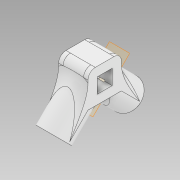
# Autodesk Inventor part: Landing_gear
Saved by Autodesk Inventor 2021 (Build 250183000, 183)
## iProperties
Created: 2020-11-24
Part Number: Landing_gear
Material: ABS Plastic
Document SubType Name: Modeling
Designer: Kanenas
Mass: 1.25971 g
Surface Area: 12.7544 cm^2
Volume: 1.1884 cm^3
Density: 1.06 g/cm^3
Appearance: Smooth - White
Author: Kanenas
Autodesk Inventor part; units mm, degrees
ref_plane "YZ Plane" through (0, 0, 0) normal (1, 0, 0) x (0, 1, 0)
ref_plane "XZ Plane" through (0, 0, 0) normal (0, 1, 0) x (-1, 0, 0)
ref_plane "XY Plane" through (0, 0, 0) normal (0, 0, 1) x (1, 0, 0)
sketch "Sketch1" plane through (0, 0, 0) normal (1, 0, 0) x (0, 1, 0)
  line L0 (2.05, 2.05) -> (-2.05, 2.05)
  line L1 (-2.05, 2.05) -> (-2.05, -2.05)
  line L2 (-2.05, -2.05) -> (2.05, -2.05)
  line L3 (2.05, -2.05) -> (2.05, 2.05)
  line L4 (2.05, 2.05) -> (-2.05, -2.05) construction
  line L5 (-2.05, 2.05) -> (2.05, -2.05) construction
  line L6 (4.55, 4.55) -> (-4.55, 4.55)
  line L7 (-4.55, 4.55) -> (-4.55, -4.55)
  line L8 (-4.55, -4.55) -> (4.55, -4.55)
  line L9 (4.55, -4.55) -> (4.55, 4.55)
  line L10 (4.55, 4.55) -> (-4.55, -4.55) construction
  line L11 (-4.55, 4.55) -> (4.55, -4.55) construction
  point P0 (0, 0)
  dimension "d0" = 4.1
  dimension "d1" = 4.1
  dimension "d2" = 9.1
  dimension "d3" = 9.1
  constraints: 24 end point, 4 midpoint, 4 parallel, 2 horizontal, 2 perpendicular
  measures "d0" distance of L2.end L0.start
  measures "d1" distance of L1.end L2.end
  measures "d2" distance of L8.end L6.start
  measures "d3" distance of L7.end L8.end
extrude "Extrusion1" add sketch "Sketch1" along normal blind 8
ref_plane "Work Plane1" through (0, -4.55, -4.55) normal (0, 0.7071068, 0.7071068) x (1, 0, 0)
sketch "Sketch2" plane through (0, -4.55, -4.55) normal (0, 0.7071068, 0.7071068) x (1, 0, 0)
  line L0 (0, 0) -> (8, 0) projected
  circle A0 centre (4, 0) radius 4
  circle A1 centre (4, 0) radius 2.05
  dimension "d7" = 8
  dimension "d8" = 4.1
  constraints: 2 centre point, 1 coincident, 1 midpoint
  measures "d7" diameter of A0
  measures "d8" diameter of A1
extrude "Extrusion2" add sketch "Sketch2" along normal mid plane 15 contours A1 L0 A0 | L0 A0 A1
mirror "Mirror1" about plane through (0, 0, 0) normal (0, 0, 1) of "Extrusion2"
sketch "Sketch3" plane through (8, 0, 0) normal (1, 0, 0) x (0, 0, -1)
  line L0 (-2.05, 2.05) -> (2.05, 2.05) projected
  line L1 (-2.05, -2.05) -> (-2.05, 2.05) projected
  line L2 (2.05, -2.05) -> (-2.05, -2.05) projected
  line L3 (2.05, 2.05) -> (2.05, -2.05) projected
  point P0 (0, 0)
extrude "Extrusion3" cut sketch "Sketch3" against normal blind 10
sketch "Sketch4" plane through (4, -9.8533, 9.8533) normal (0, -0.7071068, 0.7071068) x (1, 0, 0)
  circle A0 centre (0, 0) radius 2 projected
  point P0 (-4, 0)
extrude "Extrusion4" cut sketch "Sketch4" against normal blind 11.25
mirror "Mirror2" about plane through (0, 0, 0) normal (0, 0, 1) of "Extrusion4"
fillet "Fillet2" radius 5 4 edges at (5.2511, -5.373, 0) (2.7489, -5.373, 0) (4, 1.1069, 4.55) (4, 1.1069, -4.55)
fillet "Fillet3" radius 2 2 edges at (4, 4.55, 4.55) (4, 4.55, -4.55)
equation "\"d3\" = d2"
body "Solid1"
